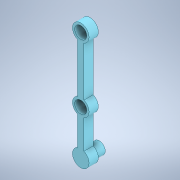
# Autodesk Inventor part: Component27
Saved by Autodesk Inventor 2022 (Build 260153000, 153)
## iProperties
Created: 2022-01-29
Part Number: Component27
Material: Generic
Document SubType Name: Modeling
Designer: Administrator
Density: 1 g/cm^3
Appearance: Default
Title: Component27
Author: Administrator
Autodesk Inventor part; units mm, degrees
ref_plane "YZ Plane" through (0, 0, 0) normal (1, 0, 0) x (0, 1, 0)
ref_plane "XZ Plane" through (0, 0, 0) normal (0, 1, 0) x (-1, 0, 0)
ref_plane "XY Plane" through (0, 0, 0) normal (0, 0, 1) x (1, 0, 0)
sketch "Sketch2" plane through (0, 0, 0) normal (0, 0, 1) x (1, 0, 0)
  circle A0 centre (0, -32.6543) radius 3.25
  circle A1 centre (0, 26.3457) radius 3.25
  circle A2 centre (0, -8.6543) radius 3.25
  line L0 (-1.7446, -4.5062) -> (-1.7446, 22.1977)
  arc A3 (1.7446, 22.1977) -> (-1.7446, 22.1977) centre (0, 26.3457) ccw
  arc A4 (1.7446, -12.8023) -> (1.7446, -4.5062) centre (0, -8.6543) ccw
  arc A5 (-1.7446, -28.5062) -> (1.7446, -28.5062) centre (0, -32.6543) ccw
  line L1 (-1.7446, -28.5062) -> (-1.7446, -12.8023)
  arc A6 (-1.7446, -4.5062) -> (-1.7446, -12.8023) centre (0, -8.6543) ccw
  line L2 (0, 47.7105) -> (0, -62.3205) construction
  line L3 (1.7446, -4.5062) -> (1.7446, 22.1977)
  line L4 (1.7446, -28.5062) -> (1.7446, -12.8023)
  point P0 (0, 0)
  dimension "d4" = 6.5
  dimension "d5" = 24
  dimension "d6" = 35
  dimension "d8" = 9
  constraints: 10 end point, 8 point on circle, 7 centre point, 5 equal radius, 4 coincident, 4 symmetric about line, 2 point on line, 2 vertical, 1 collinear
  measures "d4" diameter of A2
  measures "d5" distance of A2.centre A0.centre
  measures "d6" distance of A1.centre A2.centre
  measures "d8" diameter of A3
extrude "Extrusion1" add sketch "Sketch2" along normal blind 5 contours A0 | L0 A3 L3 A4 L4 A5 L1 A6
extrude "Extrusion2" add sketch "Sketch2" against normal blind 5 contours A0
equation "\"d4\" = R"
equation "\"d8\" = R1"
equation "\"d0\" = thickness"
equation "\"R\" = 6.5"
equation "\"thickness\" = 5"
equation "\"width\" = 6.5"
equation "\"R1\" = 9"
body "Solid1"
